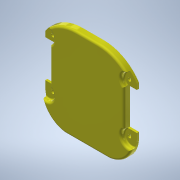
# Autodesk Inventor part: coque_inf
Saved by Autodesk Inventor 2021 (Build 250183000, 183)
## iProperties
Created: 2015-03-17
Part Number: coque_inf
Material: Plastique ABS
Document SubType Name: Modeling
Designer: sd
Density: 1.06 g/cm^3
Appearance: Lisse - Jaune
Mass: 14.9206 g
Surface Area: 155.307 cm^2
Volume: 14.0761 cm^3
Author: sd
Autodesk Inventor part; units mm, degrees
ref_plane "YZ Plane" through (0, 0, 0) normal (1, 0, 0) x (0, 1, 0)
ref_plane "XZ Plane" through (0, 0, 0) normal (0, 1, 0) x (-1, 0, 0)
ref_plane "XY Plane" through (0, 0, 0) normal (0, 0, 1) x (1, 0, 0)
sketch "Esquisse1" plane through (0, 0, 0) normal (0, 1, 0) x (-1, 0, 0)
  line L0 (-43, -44) -> (43, -44)
  line L1 (43, -44) -> (43, 44)
  line L2 (43, 44) -> (-43, 44)
  line L3 (-43, 44) -> (-43, -44)
  point P0 (0, 0)
  dimension "d0" = 86
  dimension "d1" = 88
  dimension "d2" = 43
  dimension "d3" = 44
  constraints: 8 end point, 2 parallel, 1 horizontal, 1 perpendicular
  measures "d0" distance of L1.end L2.end
  measures "d1" distance of L2.end L0.start
  measures "d2" horizontal distance of point (0, 0) L2.end
  measures "d3" vertical distance of point (0, 0) L2.end
extrude "Carre de base" add sketch "Esquisse1" along normal blind 6
sketch "Esquisse2" plane through (0, 6, 0) normal (0, 1, 0) x (1, 0, 0)
  line L0 (43, 44) -> (-43, 44) projected
  line L1 (-43, 44) -> (-43, -44) projected
  line L2 (-43, -44) -> (43, -44) projected
  line L3 (43, -44) -> (43, 44) projected
  line L4 (-43, 14) -> (-34.5, 14)
  line L5 (-34.5, 14) -> (-34.5, -21)
  line L6 (-34.5, -21) -> (-43, -21)
  line L7 (43, 14) -> (34.5, 14)
  line L8 (34.5, 14) -> (34.5, -21)
  line L9 (34.5, -21) -> (43, -21)
  line L10 (-43, -21) -> (-43, -26)
  line L11 (43, -21) -> (43, -26)
  line L12 (-43, 14) -> (-43, 19)
  line L13 (43, 14) -> (43, 19)
  line L14 (10, -44) -> (-10, -44)
  line L15 (21, 44) -> (-21, 44)
  arc A0 (10, -44) -> (43, -26) centre (10, -4.75) ccw
  arc A1 (-43, -26) -> (-10, -44) centre (-10, -4.75) ccw
  arc A2 (43, 19) -> (21, 44) centre (17.7955, 19) ccw
  arc A3 (-21, 44) -> (-43, 19) centre (-17.7955, 19) ccw
  point P0 (0, 0)
  dimension "d6" = 35
  dimension "d7" = 30
  dimension "d8" = 30
  dimension "d9" = 8.5
  dimension "d10" = 8.5
  dimension "d11" = 35
  dimension "d13" = 5
  dimension "d14" = 5
  dimension "d15" = 5
  dimension "d16" = 5
  dimension "d21" = 20
  dimension "d22" = 10
  dimension "d23" = 42
  dimension "d24" = 21
  dimension "d25" = 39.25
  dimension "d26" = 39.25
  dimension "d27" = 25.2046
  dimension "d28" = 25.2046
  constraints: 24 end point, 12 point on line, 8 point on circle, 4 centre point, 4 perpendicular, 2 parallel, 2 tangent
  measures "d6" distance of L4.end L5.end
  measures "d7" distance from line of L0 L4.end
  measures "d8" distance between parallel lines of L0 L7
  measures "d9" distance of L7.start L7.end
  measures "d10" distance of L4.start L4.end
  measures "d11" distance of L7.end L8.end
  measures "d13" distance of L9.end L11.end
  measures "d14" distance of L6.end L10.end
  measures "d15" distance of L7.start L13.end
  measures "d16" distance of L4.start L12.end
  measures "d21" distance of L14.start L14.end
  measures "d22" horizontal distance of point (0, 0) L14.start
  measures "d23" distance of L15.start L15.end
  measures "d24" horizontal distance of point (0, 0) L15.start
  measures "d25" radius of A0
  measures "d26" radius of A1
  measures "d27" radius of A2
  measures "d28" radius of A3
extrude "Evidement" cut sketch "Esquisse2" against normal through all contours L3 A2 L0 | A3 L1 L0 | L3 L9 L8 L7 | L4 L5 L6 L1 | L3 L2 A0 | A1 L2 L1
sketch "Esquisse9" plane through (0, 0, 0) normal (0, -1, 0) x (1, 0, 0)
  circle A0 centre (36, 26) radius 1.6
  circle A1 centre (36, -20) radius 1.6
  circle A2 centre (-36, -20) radius 1.6
  circle A3 centre (-36, 26) radius 1.6
  point P0 (0, 0)
  dimension "d86" = 3.2
  dimension "d87" = 3.2
  dimension "d88" = 3.2
  dimension "d89" = 3.2
  dimension "d90" = 36
  dimension "d91" = 36
  dimension "d92" = 36
  dimension "d93" = 36
  dimension "d94" = 20
  dimension "d95" = 20
  dimension "d96" = 26
  dimension "d97" = 26
  constraints: 4 centre point
  measures "d86" diameter of A0
  measures "d87" diameter of A1
  measures "d88" diameter of A3
  measures "d89" diameter of A2
  measures "d90" horizontal distance of point (0, 0) A3.centre
  measures "d91" horizontal distance of point (0, 0) A0.centre
  measures "d92" horizontal distance of point (0, 0) A1.centre
  measures "d93" horizontal distance of point (0, 0) A2.centre
  measures "d94" vertical distance of point (0, 0) A2.centre
  measures "d95" vertical distance of point (0, 0) A1.centre
  measures "d96" vertical distance of point (0, 0) A0.centre
  measures "d97" vertical distance of point (0, 0) A3.centre
extrude "Extrusion9" cut sketch "Esquisse9" against normal through all
sketch "Esquisse7" plane through (0, 0, 0) normal (0, -1, 0) x (1, 0, 0)
  line L0 (-34.5, -14) -> (-34.5, 21) projected
  circle A0 centre (-39, 26.5) radius 7.5
  circle A1 centre (39, 26.5) radius 7.5
  line L1 (34.5, -14) -> (43, -14) projected
  circle A2 centre (39, -19.5) radius 7.5
  line L2 (-43, -14) -> (-34.5, -14) projected
  circle A3 centre (-39, -19.5) radius 7.5
  point P0 (0, 0)
  dimension "d74" = 15
  dimension "d75" = 15
  dimension "d76" = 15
  dimension "d77" = 15
  dimension "d78" = 26.5
  dimension "d81" = 19.5
  dimension "d103" = 26.5
  dimension "d104" = 19.5
  dimension "d105" = 39
  dimension "d106" = 39
  dimension "d107" = 39
  dimension "d108" = 39
  constraints: 4 centre point
  measures "d74" diameter of A0
  measures "d75" diameter of A1
  measures "d76" diameter of A3
  measures "d77" diameter of A2
  measures "d78" vertical distance of point (0, 0) A0.centre
  measures "d81" vertical distance of point (0, 0) A3.centre
  measures "d103" vertical distance of point (0, 0) A1.centre
  measures "d104" vertical distance of point (0, 0) A2.centre
  measures "d105" horizontal distance of point (0, 0) A1.centre
  measures "d106" horizontal distance of point (0, 0) A2.centre
  measures "d107" horizontal distance of point (0, 0) A0.centre
  measures "d108" horizontal distance of point (0, 0) A3.centre
extrude "Extrusion8" cut sketch "Esquisse7" against normal blind 4
fillet "Congé2" radius 2 12 edges at (0, 0, 44) (-24.2814, 0, 41.3096) (24.2814, 0, 41.3096) (31.5949, 0, 27.6892) (34.5, 0, 3.5) (32.4874, 0, -23.2197) (34.0258, 0, -38.2833) (0, 0, -44) (-34.0258, 0, -38.2833) (-32.4874, 0, -23.2197) (-34.5, 0, 3.5) (-31.5949, 0, 27.6892)
fillet "Congé3" radius 1 4 edges at (31.5949, 4, 27.6892) (32.4874, 4, -23.2197) (-32.4874, 4, -23.2197) (-31.5949, 4, 27.6892)
shell "Coque3" thickness 1.9 removed faces 1 at (11.5, 6, 9.3333)
equation "\"d2\" = 0.5 * d0"
equation "\"d3\" = 0.5 * d1"
equation "\"d8\" = d7"
equation "\"d9\" = d10"
equation "\"d11\" = d6"
equation "\"d13\" = d14"
equation "\"d15\" = d16"
equation "\"d22\" = 0.5 * d21"
equation "\"d24\" = 0.5 * d23"
equation "\"d26\" = d25"
equation "\"d28\" = d27"
equation "\"d88\" = d86"
equation "\"d89\" = d86"
equation "\"d91\" = d90"
equation "\"d92\" = d90"
equation "\"d93\" = d90"
equation "\"d95\" = d94"
equation "\"d97\" = d96"
equation "\"d74\" = d75"
equation "\"d75\" = d77"
equation "\"d76\" = d74"
equation "\"d78\" = d103"
equation "\"d81\" = d80"
equation "\"d106\" = d105"
equation "\"d107\" = d105"
equation "\"d108\" = d105"
equation "\"d80\" = 19.5"
